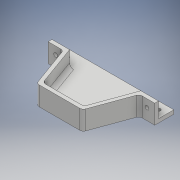
# Autodesk Inventor part: エンコーダガード2
Saved by Autodesk Inventor 2017 (Build 210142000, 142)
## iProperties
Part Number: エンコーダガード2
Material: 一般
Document SubType Name: Modeling
Designer: highs
Density: 1 g/cm^3
Appearance: 既定
Author: highs
## iProperties of the stored document エンコーダガード2_3D プリント.ipt
Part Number: エンコーダガード2_3D プリント
Material: 一般
Document SubType Name: Modeling
Designer: highs
Density: 1 g/cm^3
Appearance: 既定
Author: highs
Autodesk Inventor part; units mm, degrees
ref_plane "YZ Plane" through (0, 0, 0) normal (1, 0, 0) x (0, 1, 0)
ref_plane "XZ Plane" through (0, 0, 0) normal (0, 1, 0) x (-1, 0, 0)
ref_plane "XY Plane" through (0, 0, 0) normal (0, 0, 1) x (1, 0, 0)
sketch "スケッチ1" plane through (0, 0, 0) normal (0, 0, 1) x (1, 0, 0)
  line L0 (0, 0) -> (0, -25)
  line L1 (0, -25) -> (20, -25)
  line L2 (20, -25) -> (40, -80)
  line L3 (40, -80) -> (100, -80)
  line L4 (100, -80) -> (120, -25)
  line L5 (120, -25) -> (140, -25)
  line L6 (140, -25) -> (140, 0)
  line L7 (140, 0) -> (0, 0)
  line L8 (0, -20) -> (140, -20) construction
  line L9 (0, -10) -> (140, -10) construction
  circle A0 centre (10, -10) radius 2.5
  circle A1 centre (130, -10) radius 2.5
  dimension "d14" = 20
  dimension "d15" = 25
  dimension "d16" = 140
  dimension "d17" = 20
  dimension "d18" = 60
  dimension "d19" = 60
  dimension "d20" = 5
  dimension "d21" = 10
  dimension "d22" = 10
  dimension "d23" = 10
  constraints: 20 end point, 8 point on line, 5 perpendicular, 2 centre point, 2 equal length, 1 equal radius, 1 parallel, 1 vertical
  measures "d14" distance of L0.end L1.end
  measures "d15" distance of L0.start L0.end
  measures "d16" distance of L6.end L0.start
  measures "d17" distance between parallel lines of L7 L8
  measures "d18" distance between parallel lines of L3 L8
  measures "d19" distance of L2.end L3.end
  measures "d20" diameter of A0
  measures "d21" distance from line of L0 A0.centre
  measures "d22" distance from line of L6 A1.centre
  measures "d23" distance between parallel lines of L7 L9
extrude "押し出し3" add sketch "スケッチ1" along normal blind 5
sketch "スケッチ3" plane through (0, 0, 5) normal (0, 0, 1) x (1, 0, 0)
  line L0 (0, 0) -> (0, -25) projected
  line L1 (0, -20) -> (0, -25)
  line L2 (0, -25) -> (20, -25) projected
  line L3 (0, -25) -> (20, -25)
  line L4 (20, -25) -> (40, -80) projected
  line L5 (20, -25) -> (40, -80)
  line L6 (40, -80) -> (100, -80) projected
  line L7 (40, -80) -> (100, -80)
  line L8 (120, -25) -> (140, -25) projected
  line L9 (100, -80) -> (120, -25)
  line L10 (120, -25) -> (140, -25)
  line L11 (140, -25) -> (140, 0)
  line L12 (140, -25) -> (140, -20)
  line L13 (140, -20) -> (116.8182, -20)
  line L14 (116.8182, -20) -> (96.8182, -75)
  line L15 (96.8182, -75) -> (43.1818, -75)
  line L16 (43.1818, -75) -> (23.1818, -20)
  line L17 (23.1818, -20) -> (0, -20)
  line L18 (100, -80) -> (120, -25) projected
  line L19 (43.1818, -75) -> (45, -80) construction
  dimension "d26" = 5
  dimension "d28" = 5
  dimension "d29" = 5
  constraints: 28 end point, 7 parallel, 5 collinear, 4 point on line, 2 horizontal, 1 perpendicular, 1 vertical
  measures "d26" distance between parallel lines of L17 L2
  measures "d28" distance of L4.end L19.end
  measures "d29" distance between parallel lines of L6 L15
extrude "押し出し4" add sketch "スケッチ3" along normal blind 20
sketch "スケッチ4" plane through (116.8182, -20, 5) normal (0, 1, 0) x (1, 0, 0)
  line L0 (23.1818, 5) -> (23.1818, -20) construction
  line L1 (23.1818, -10) -> (-116.4286, -10) construction
  line L2 (23.1818, -20) -> (0, -20) construction
  circle A0 centre (13.1818, -10) radius 2.5
  circle A1 centre (-106.8182, -10) radius 2.5
  line L3 (-116.8182, 0) -> (-116.8182, -20) construction
  point P0 (-116.8182, 5)
  dimension "d32" = 10
  dimension "d33" = 10
  dimension "d34" = 5
  dimension "d35" = 10
  constraints: 3 point on line, 2 centre point, 2 end point, 1 equal radius, 1 horizontal
  measures "d32" distance between parallel lines of L2 L1
  measures "d33" distance from line of L0 A0.centre
  measures "d34" diameter of A0
  measures "d35" distance from line of L3 A1.centre
extrude "押し出し5" cut sketch "スケッチ4" against normal blind 20
fillet "フィレット1" radius 5 3 edges at (33.1818, -47.5, 5) (70, -75, 5) (106.8182, -47.5, 5)
fillet "フィレット1" radius 5 6 edges at (20, -25, 12.5) (120, -25, 12.5) (43.1818, -75, 15) (96.8182, -75, 15) (40, -80, 12.5) (100, -80, 12.5)
